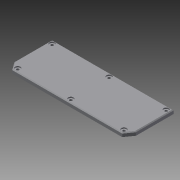
# Autodesk Inventor part: panel plain
Saved by Autodesk Inventor 2014 (Build 180170000, 170)
## iProperties
Created: 2015-02-26
Part Number: panel plain
Material: Generic
Document SubType Name: Modeling
Designer: james_III
Density: 1 g/cm^3
Appearance: Default
Author: james_III
Autodesk Inventor part; units mm, degrees
ref_plane "YZ Plane" through (0, 0, 0) normal (1, 0, 0) x (0, 1, 0)
ref_plane "XZ Plane" through (0, 0, 0) normal (0, 1, 0) x (-1, 0, 0)
ref_plane "XY Plane" through (0, 0, 0) normal (0, 0, 1) x (1, 0, 0)
sketch "Sketch1" plane through (0, 0, 0) normal (0, 0, 1) x (1, 0, 0)
  line L0 (-75.9981, -21.58) -> (-77.5, -19.4559) projected
  line L1 (-77.5, -19.4559) -> (-77.5, 17.5699) projected
  arc A0 (-75.5, 19.5699) -> (-77.5, 17.5699) centre (-75.5, 17.5699) ccw projected
  arc A1 (-75.5, 19.5699) -> (-70.5, 24.5699) centre (-75.5, 24.5699) ccw projected
  arc A2 (-68.5, 26.5699) -> (-70.5, 24.5699) centre (-68.5, 24.5699) ccw projected
  line L2 (-68.5, 26.5699) -> (-7, 26.5699) projected
  arc A3 (-5, 24.5699) -> (-7, 26.5699) centre (-7, 24.5699) ccw projected
  arc A4 (-5, 24.5699) -> (5, 24.5699) centre (0, 24.5699) ccw projected
  arc A5 (7, 26.5699) -> (5, 24.5699) centre (7, 24.5699) ccw projected
  line L3 (7, 26.5699) -> (68.5, 26.5699) projected
  arc A6 (70.5, 24.5699) -> (68.5, 26.5699) centre (68.5, 24.5699) ccw projected
  arc A7 (70.5, 24.5699) -> (75.5, 19.5699) centre (75.5, 24.5699) ccw projected
  arc A8 (77.5, 17.5699) -> (75.5, 19.5699) centre (75.5, 17.5699) ccw projected
  line L4 (77.5, 17.5699) -> (77.5, -19.4559) projected
  line L5 (77.5, -19.4559) -> (75.9981, -21.58) projected
  arc A9 (73.2104, -22.0583) -> (75.9981, -21.58) centre (74.3651, -20.4253) ccw projected
  arc A10 (73.2104, -22.0583) -> (65.3236, -26.1408) centre (70.3236, -26.1408) ccw projected
  arc A11 (63.3236, -28.1408) -> (65.3236, -26.1408) centre (63.3236, -26.1408) ccw projected
  line L6 (63.3236, -28.1408) -> (7, -28.1408) projected
  arc A12 (5, -26.1408) -> (7, -28.1408) centre (7, -26.1408) ccw projected
  arc A13 (5, -26.1408) -> (-5, -26.1408) centre (0, -26.1408) ccw projected
  arc A14 (-7, -28.1408) -> (-5, -26.1408) centre (-7, -26.1408) ccw projected
  line L7 (-7, -28.1408) -> (-63.3236, -28.1408) projected
  arc A15 (-65.3236, -26.1408) -> (-63.3236, -28.1408) centre (-63.3236, -26.1408) ccw projected
  arc A16 (-65.3236, -26.1408) -> (-73.2104, -22.0583) centre (-70.3236, -26.1408) ccw projected
  arc A17 (-75.9981, -21.58) -> (-73.2104, -22.0583) centre (-74.3651, -20.4253) ccw projected
  circle A18 centre (70.3236, -26.1408) radius 1.25 projected
  circle A19 centre (0, 24.5699) radius 1.25 projected
  circle A20 centre (-70.3236, -26.1408) radius 1.25 projected
  circle A21 centre (-75.5, 24.5699) radius 1.25 projected
  circle A22 centre (75.5, 24.5699) radius 1.25 projected
  circle A23 centre (0, -26.1408) radius 1.25 projected
  line L8 (-80.5, -20.4094) -> (-80.5, 29.5699) projected
  line L9 (-72.9118, -31.1408) -> (-80.5, -20.4094) projected
  line L10 (72.9118, -31.1408) -> (-72.9118, -31.1408) projected
  line L11 (80.5, -20.4094) -> (72.9118, -31.1408) projected
  line L12 (80.5, 29.5699) -> (80.5, -20.4094) projected
  line L13 (-80.5, 29.5699) -> (80.5, 29.5699) projected
  line L14 (-72.8342, -30.9908) -> (-80.35, -20.3618)
  line L15 (-80.35, -20.3618) -> (-80.35, 29.4199)
  line L16 (-80.35, 29.4199) -> (80.35, 29.4199)
  line L17 (80.35, 29.4199) -> (80.35, -20.3618)
  line L18 (80.35, -20.3618) -> (72.8342, -30.9908)
  line L19 (72.8342, -30.9908) -> (-72.8342, -30.9908)
  point P0 (0, 0)
  dimension "d0" = 0.15
  constraints: 12 end point, 5 other
  measures "d0" distance between parallel lines of L10 L19
extrude "Extrusion1" add sketch "Sketch1" along normal blind 5 contours L0 L1 A0 A1 A2 L2 A3 A4 A5 L3 A6 A7 A8 L4 L5 A9 A10 A11 L6 A12 A13 A14 L7 A15 A16 A17 | L14 L15 L16 L17 L18 L19
sketch "Sketch2" plane through (0, 0, 5) normal (0, 0, 1) x (1, 0, 0)
  circle A0 centre (0, -26.1408) radius 1.25 projected
  circle A1 centre (75.5, 24.5699) radius 1.25 projected
  circle A2 centre (-75.5, 24.5699) radius 1.25 projected
  circle A3 centre (-70.3236, -26.1408) radius 1.25 projected
  circle A4 centre (0, 24.5699) radius 1.25 projected
  circle A5 centre (70.3236, -26.1408) radius 1.25 projected
  point P0 (0, 0)
  constraints: 6 coincident
hole "Hole1" at (-75.5, 24.5699, 5) at (0, 24.5699, 5) at (75.5, 24.5699, 5) at (70.3236, -26.1408, 5) at (0, -26.1408, 5) at (-70.3236, -26.1408, 5) direction (0, 0, -1) diameter 3.5 depth 8 tip angle 118 counterbore diameter 7 counterbore depth 1.5
chamfer "Chamfer1" distance 1 angle 45 6 edges at (0, -30.9908, 5) (76.5921, -25.6763, 5) (80.35, 4.5291, 5) (0, 29.4199, 5) (-80.35, 4.5291, 5) (-76.5921, -25.6763, 5)
body "Solid1"
